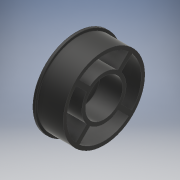
# Autodesk Inventor part: 바퀴8PI
Saved by Autodesk Inventor 2017 (Build 210142000, 142)
## iProperties
Part Number: 바퀴8PI
Material: 아세탈 수지, 검은색
Document SubType Name: Modeling
Designer: minom
Density: 1.425 g/cm^3
Appearance: 매끄러움 - 검은색
Author: minom
Autodesk Inventor part; units mm, degrees
ref_plane "YZ Plane" through (0, 0, 0) normal (1, 0, 0) x (0, 1, 0)
ref_plane "XZ Plane" through (0, 0, 0) normal (0, 1, 0) x (-1, 0, 0)
ref_plane "XY Plane" through (0, 0, 0) normal (0, 0, 1) x (1, 0, 0)
sketch "스케치1" plane through (0, 0, 0) normal (1, 0, 0) x (0, 1, 0)
  circle A0 centre (0, 0) radius 37
  circle A1 centre (0, 0) radius 4
  dimension "d0" = 74
  dimension "d1" = 8
  constraints: 2 centre point, 2 coincident
  measures "d0" diameter of A0
  measures "d1" diameter of A1
extrude "돌출1" add sketch "스케치1" along normal blind 24
sketch "스케치2" plane through (24, 0, 0) normal (1, 0, 0) x (0, 0, -1)
  circle A0 centre (0, 0) radius 16
  dimension "d4" = 32
  constraints: 1 centre point, 1 coincident
  measures "d4" diameter of A0
extrude "돌출2" cut sketch "스케치2" against normal blind 19
sketch "스케치4" plane through (5, 0, 0) normal (1, 0, 0) x (0, 0, -1)
  circle A0 centre (0, 10) radius 1.75
  circle A1 centre (10, 0) radius 1.75
  circle A2 centre (0, -10) radius 1.75
  circle A3 centre (-10, 0) radius 1.75
  point P0 (0, 0)
  dimension "d8" = 3.5
  dimension "d9" = 3.5
  dimension "d10" = 3.5
  dimension "d11" = 3.5
  constraints: 4 centre point
  measures "d8" diameter of A0
  measures "d9" diameter of A1
  measures "d10" diameter of A2
  measures "d11" diameter of A3
extrude "돌출3" cut sketch "스케치4" against normal blind 19
sketch "스케치5" plane through (24, 0, 0) normal (1, 0, 0) x (0, 0, -1)
  circle A0 centre (0, 0) radius 19
  circle A1 centre (0, 0) radius 32
  line L0 (-19.4142, 16.5858) -> (-14.7746, 11.9462)
  line L1 (-23.9974, 21.169) -> (-19.4142, 16.5858)
  line L2 (-16.5858, 19.4142) -> (-11.9462, 14.7746)
  line L3 (-16.5858, 19.4142) -> (-21.169, 23.9974)
  line L4 (16.5858, 19.4142) -> (11.9462, 14.7746)
  line L5 (16.5858, 19.4142) -> (21.169, 23.9974)
  line L6 (19.4142, 16.5858) -> (23.9974, 21.169)
  line L7 (19.4142, 16.5858) -> (14.7746, 11.9462)
  line L8 (16.5858, -19.4142) -> (11.9462, -14.7746)
  line L9 (16.5858, -19.4142) -> (21.169, -23.9974)
  line L10 (19.4142, -16.5858) -> (14.7746, -11.9462)
  line L11 (19.4142, -16.5858) -> (23.9974, -21.169)
  line L12 (-19.4142, -16.5858) -> (-14.7746, -11.9462)
  line L13 (-19.4142, -16.5858) -> (-23.9974, -21.169)
  line L14 (-16.5858, -19.4142) -> (-11.9462, -14.7746)
  line L15 (-16.5858, -19.4142) -> (-21.169, -23.9974)
  line L16 (-14.7746, -11.9462) -> (-23.9974, -21.169)
  dimension "d18" = 4
  constraints: 34 end point, 13 point on line, 1 coincident, 1 collinear, 1 parallel, 20 other
  measures "d18" distance of L2.start L0.start
extrude "돌출4" cut sketch "스케치5" against normal blind 19 contours A0 L7 L6 A1 L11 L10 | A0 L2 L3 A1 L5 L4 | L8 L9 A1 L15 L14 A0 | A0 L12 L13 A1 L1 L0
sketch "스케치6" plane through (24, 0, 0) normal (1, 0, 0) x (0, 0, -1)
  circle A0 centre (0, 0) radius 35
  circle A1 centre (0, 0) radius 37
  dimension "d22" = 70
  constraints: 2 centre point, 2 coincident
  measures "d22" diameter of A0
extrude "돌출5" cut sketch "스케치6" against normal blind 22
